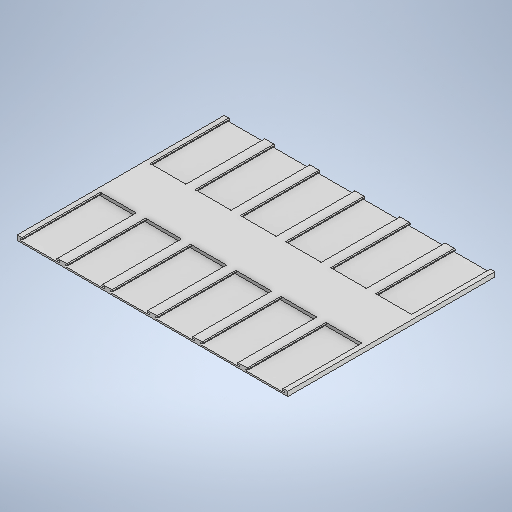
# Autodesk Inventor part: Holder
Saved by Autodesk Inventor 2025 (Build 290162000, 162)
## iProperties
Created: 2025-01-15
Part Number: Holder
Material: Generic
Document SubType Name: Modeling
Designer: ethan
Density: 1 g/cm^3
Appearance: Default
Author: ethan
Autodesk Inventor part; units mm, degrees
ref_plane "YZ Plane" through (0, 0, 0) normal (1, 0, 0) x (0, 1, 0)
ref_plane "XZ Plane" through (0, 0, 0) normal (0, 1, 0) x (-1, 0, 0)
ref_plane "XY Plane" through (0, 0, 0) normal (0, 0, 1) x (1, 0, 0)
sketch "Sketch1" plane through (0, 0, 0) normal (0, 1, 0) x (-1, 0, 0)
  line L0 (0, 0) -> (25.4, 0) construction
  line L1 (25.4, 0) -> (25.4, -50.8) construction
  line L2 (25.4, -50.8) -> (0, -50.8) construction
  line L3 (0, -50.8) -> (0, 0) construction
  line L4 (23.9, -49.3) -> (23.9, -1.5) construction
  line L5 (23.9, -1.5) -> (1.5, -1.5) construction
  line L6 (1.5, -1.5) -> (1.5, -49.3) construction
  line L7 (1.5, -49.3) -> (23.9, -49.3) construction
  line L8 (0, 0) -> (-4, 0) construction
  line L9 (-29.4, 0) -> (-4, 0) construction
  line L10 (-4, 0) -> (-4, -50.8) construction
  line L11 (-4, -50.8) -> (-29.4, -50.8) construction
  line L12 (-29.4, -50.8) -> (-29.4, 0) construction
  line L13 (-5.5, -49.3) -> (-5.5, -1.5) construction
  line L14 (-5.5, -1.5) -> (-27.9, -1.5) construction
  line L15 (-27.9, -1.5) -> (-27.9, -49.3) construction
  line L16 (-27.9, -49.3) -> (-5.5, -49.3) construction
  line L17 (-58.8, 0) -> (-33.4, 0) construction
  line L18 (-33.4, 0) -> (-33.4, -50.8) construction
  line L19 (-33.4, -50.8) -> (-58.8, -50.8) construction
  line L20 (-58.8, -50.8) -> (-58.8, 0) construction
  line L21 (-34.9, -49.3) -> (-34.9, -1.5) construction
  line L22 (-34.9, -1.5) -> (-57.3, -1.5) construction
  line L23 (-57.3, -1.5) -> (-57.3, -49.3) construction
  line L24 (-57.3, -49.3) -> (-34.9, -49.3) construction
  line L25 (-88.2, 0) -> (-62.8, 0) construction
  line L26 (-62.8, 0) -> (-62.8, -50.8) construction
  line L27 (-62.8, -50.8) -> (-88.2, -50.8) construction
  line L28 (-88.2, -50.8) -> (-88.2, 0) construction
  line L29 (-64.3, -49.3) -> (-64.3, -1.5) construction
  line L30 (-64.3, -1.5) -> (-86.7, -1.5) construction
  line L31 (-86.7, -1.5) -> (-86.7, -49.3) construction
  line L32 (-86.7, -49.3) -> (-64.3, -49.3) construction
  line L33 (-117.6, 0) -> (-92.2, 0) construction
  line L34 (-92.2, 0) -> (-92.2, -50.8) construction
  line L35 (-92.2, -50.8) -> (-117.6, -50.8) construction
  line L36 (-117.6, -50.8) -> (-117.6, 0) construction
  line L37 (-93.7, -49.3) -> (-93.7, -1.5) construction
  line L38 (-93.7, -1.5) -> (-116.1, -1.5) construction
  line L39 (-116.1, -1.5) -> (-116.1, -49.3) construction
  line L40 (-116.1, -49.3) -> (-93.7, -49.3) construction
  line L41 (-147, 0) -> (-121.6, 0) construction
  line L42 (-121.6, 0) -> (-121.6, -50.8) construction
  line L43 (-121.6, -50.8) -> (-147, -50.8) construction
  line L44 (-147, -50.8) -> (-147, 0) construction
  line L45 (-123.1, -49.3) -> (-123.1, -1.5) construction
  line L46 (-123.1, -1.5) -> (-145.5, -1.5) construction
  line L47 (-145.5, -1.5) -> (-145.5, -49.3) construction
  line L48 (-145.5, -49.3) -> (-123.1, -49.3) construction
  line L49 (0, 80.2) -> (25.4, 80.2) construction
  line L50 (25.4, 80.2) -> (25.4, 29.4) construction
  line L51 (25.4, 29.4) -> (0, 29.4) construction
  line L52 (0, 29.4) -> (0, 80.2) construction
  line L53 (23.9, 30.9) -> (23.9, 78.7) construction
  line L54 (23.9, 78.7) -> (1.5, 78.7) construction
  line L55 (1.5, 78.7) -> (1.5, 30.9) construction
  line L56 (1.5, 30.9) -> (23.9, 30.9) construction
  line L57 (-29.4, 80.2) -> (-4, 80.2) construction
  line L58 (-4, 80.2) -> (-4, 29.4) construction
  line L59 (-4, 29.4) -> (-29.4, 29.4) construction
  line L60 (-29.4, 29.4) -> (-29.4, 80.2) construction
  line L61 (-5.5, 30.9) -> (-5.5, 78.7) construction
  line L62 (-5.5, 78.7) -> (-27.9, 78.7) construction
  line L63 (-27.9, 78.7) -> (-27.9, 30.9) construction
  line L64 (-27.9, 30.9) -> (-5.5, 30.9) construction
  line L65 (-58.8, 80.2) -> (-33.4, 80.2) construction
  line L66 (-33.4, 80.2) -> (-33.4, 29.4) construction
  line L67 (-33.4, 29.4) -> (-58.8, 29.4) construction
  line L68 (-58.8, 29.4) -> (-58.8, 80.2) construction
  line L69 (-34.9, 30.9) -> (-34.9, 78.7) construction
  line L70 (-34.9, 78.7) -> (-57.3, 78.7) construction
  line L71 (-57.3, 78.7) -> (-57.3, 30.9) construction
  line L72 (-57.3, 30.9) -> (-34.9, 30.9) construction
  line L73 (-88.2, 80.2) -> (-62.8, 80.2) construction
  line L74 (-62.8, 80.2) -> (-62.8, 29.4) construction
  line L75 (-62.8, 29.4) -> (-88.2, 29.4) construction
  line L76 (-88.2, 29.4) -> (-88.2, 80.2) construction
  line L77 (-64.3, 30.9) -> (-64.3, 78.7) construction
  line L78 (-64.3, 78.7) -> (-86.7, 78.7) construction
  line L79 (-86.7, 78.7) -> (-86.7, 30.9) construction
  line L80 (-86.7, 30.9) -> (-64.3, 30.9) construction
  line L81 (-117.6, 80.2) -> (-92.2, 80.2) construction
  line L82 (-92.2, 80.2) -> (-92.2, 29.4) construction
  line L83 (-92.2, 29.4) -> (-117.6, 29.4) construction
  line L84 (-117.6, 29.4) -> (-117.6, 80.2) construction
  line L85 (-93.7, 30.9) -> (-93.7, 78.7) construction
  line L86 (-93.7, 78.7) -> (-116.1, 78.7) construction
  line L87 (-116.1, 78.7) -> (-116.1, 30.9) construction
  line L88 (-116.1, 30.9) -> (-93.7, 30.9) construction
  line L89 (-147, 80.2) -> (-121.6, 80.2) construction
  line L90 (-121.6, 80.2) -> (-121.6, 29.4) construction
  line L91 (-121.6, 29.4) -> (-147, 29.4) construction
  line L92 (-147, 29.4) -> (-147, 80.2) construction
  line L93 (-123.1, 30.9) -> (-123.1, 78.7) construction
  line L94 (-123.1, 78.7) -> (-145.5, 78.7) construction
  line L95 (-145.5, 78.7) -> (-145.5, 30.9) construction
  line L96 (-145.5, 30.9) -> (-123.1, 30.9) construction
  line L97 (25.4, -50.8) -> (27.4, -50.8) construction
  line L98 (27.4, -50.8) -> (27.4, -52.8) construction
  line L99 (27.4, -52.8) -> (25.4, -52.8) construction
  line L100 (25.4, -52.8) -> (25.4, -50.8) construction
  line L101 (-147, 80.2) -> (-149, 80.2) construction
  line L102 (-149, 80.2) -> (-149, 82.2) construction
  line L103 (-149, 82.2) -> (-147, 82.2) construction
  line L104 (-147, 82.2) -> (-147, 80.2) construction
  line L105 (27.4, -52.8) -> (-149, -52.8)
  line L106 (-149, -52.8) -> (-149, 82.2)
  line L107 (-149, 82.2) -> (27.4, 82.2)
  line L108 (27.4, 82.2) -> (27.4, -52.8)
  line L109 (23.9, 0) -> (27.4, 0)
  line L110 (27.4, 0) -> (27.4, -52.8)
  line L111 (27.4, -52.8) -> (23.9, -52.8)
  line L112 (23.9, -52.8) -> (23.9, 0)
  line L113 (-149, -49.3) -> (-149, -52.8)
  line L114 (-149, -52.8) -> (27.4, -52.8)
  line L115 (27.4, -52.8) -> (27.4, -49.3)
  line L116 (27.4, -1.5) -> (-149, -1.5)
  line L117 (-149, -1.5) -> (-149, 30.9)
  line L118 (-149, 30.9) -> (27.4, 30.9)
  line L119 (27.4, 30.9) -> (27.4, -1.5)
  line L120 (1.5, -1.5) -> (-5.5, -1.5)
  line L121 (-5.5, -1.5) -> (-5.5, -49.3)
  line L122 (-5.5, -49.3) -> (1.5, -49.3)
  line L123 (1.5, -49.3) -> (1.5, -1.5)
  line L124 (-27.9, -49.3) -> (-34.9, -49.3)
  line L125 (-34.9, -49.3) -> (-34.9, -1.5)
  line L126 (-34.9, -1.5) -> (-27.9, -1.5)
  line L127 (-27.9, -1.5) -> (-27.9, -49.3)
  line L128 (-57.3, -1.5) -> (-64.3, -1.5)
  line L129 (-64.3, -1.5) -> (-64.3, -49.3)
  line L130 (-64.3, -49.3) -> (-57.3, -49.3)
  line L131 (-57.3, -49.3) -> (-57.3, -1.5)
  line L132 (-86.7, -49.3) -> (-93.7, -49.3)
  line L133 (-93.7, -49.3) -> (-93.7, -1.5)
  line L134 (-93.7, -1.5) -> (-86.7, -1.5)
  line L135 (-86.7, -1.5) -> (-86.7, -49.3)
  line L136 (-116.1, -1.5) -> (-123.1, -1.5)
  line L137 (-123.1, -1.5) -> (-123.1, -49.3)
  line L138 (-123.1, -49.3) -> (-116.1, -49.3)
  line L139 (-116.1, -49.3) -> (-116.1, -1.5)
  line L140 (-145.5, -49.3) -> (-149, -49.3)
  line L141 (-149, -49.3) -> (-149, -1.5)
  line L142 (-149, -1.5) -> (-145.5, -1.5)
  line L143 (-145.5, -1.5) -> (-145.5, -49.3)
  line L144 (23.9, 30.9) -> (27.4, 30.9)
  line L145 (27.4, 30.9) -> (27.4, 78.7)
  line L146 (27.4, 78.7) -> (23.9, 78.7)
  line L147 (23.9, 78.7) -> (23.9, 30.9)
  line L148 (-149, 78.7) -> (-149, 82.2)
  line L149 (-149, 82.2) -> (27.4, 82.2)
  line L150 (27.4, 82.2) -> (27.4, 78.7)
  line L151 (-145.5, 30.9) -> (-149, 30.9)
  line L152 (-149, 30.9) -> (-149, 78.7)
  line L153 (-149, 78.7) -> (-145.5, 78.7)
  line L154 (-145.5, 78.7) -> (-145.5, 30.9)
  line L155 (-123.1, 78.7) -> (-116.1, 78.7)
  line L156 (-116.1, 78.7) -> (-116.1, 30.9)
  line L157 (-116.1, 30.9) -> (-123.1, 30.9)
  line L158 (-123.1, 30.9) -> (-123.1, 78.7)
  line L159 (-93.7, 30.9) -> (-86.7, 30.9)
  line L160 (-86.7, 30.9) -> (-86.7, 78.7)
  line L161 (-86.7, 78.7) -> (-93.7, 78.7)
  line L162 (-93.7, 78.7) -> (-93.7, 30.9)
  line L163 (-64.3, 78.7) -> (-57.3, 78.7)
  line L164 (-57.3, 78.7) -> (-57.3, 30.9)
  line L165 (-57.3, 30.9) -> (-64.3, 30.9)
  line L166 (-64.3, 30.9) -> (-64.3, 78.7)
  line L167 (-34.9, 30.9) -> (-27.9, 30.9)
  line L168 (-27.9, 30.9) -> (-27.9, 78.7)
  line L169 (-27.9, 78.7) -> (-34.9, 78.7)
  line L170 (-34.9, 78.7) -> (-34.9, 30.9)
  line L171 (-5.5, 78.7) -> (1.5, 78.7)
  line L172 (1.5, 78.7) -> (1.5, 30.9)
  line L173 (1.5, 30.9) -> (-5.5, 30.9)
  line L174 (-5.5, 30.9) -> (-5.5, 78.7)
  line L175 (-145.5, 78.7) -> (-149, 78.7)
  line L176 (-149, 78.7) -> (-149, 82.2)
  line L177 (-149, 82.2) -> (-145.5, 82.2)
  line L178 (-145.5, 82.2) -> (-145.5, 78.7)
  line L179 (-123.1, 78.7) -> (-116.1, 78.7)
  line L180 (-116.1, 78.7) -> (-116.1, 82.2)
  line L181 (-116.1, 82.2) -> (-123.1, 82.2)
  line L182 (-123.1, 82.2) -> (-123.1, 78.7)
  line L183 (-93.7, 78.7) -> (-86.7, 78.7)
  line L184 (-86.7, 78.7) -> (-86.7, 82.2)
  line L185 (-86.7, 82.2) -> (-93.7, 82.2)
  line L186 (-93.7, 82.2) -> (-93.7, 78.7)
  line L187 (-64.3, 78.7) -> (-57.3, 78.7)
  line L188 (-57.3, 78.7) -> (-57.3, 82.2)
  line L189 (-57.3, 82.2) -> (-64.3, 82.2)
  line L190 (-64.3, 82.2) -> (-64.3, 78.7)
  line L191 (-34.9, 78.7) -> (-27.9, 78.7)
  line L192 (-27.9, 78.7) -> (-27.9, 82.2)
  line L193 (-27.9, 82.2) -> (-34.9, 82.2)
  line L194 (-34.9, 82.2) -> (-34.9, 78.7)
  line L195 (-5.5, 78.7) -> (1.5, 78.7)
  line L196 (1.5, 78.7) -> (1.5, 82.2)
  line L197 (1.5, 82.2) -> (-5.5, 82.2)
  line L198 (-5.5, 82.2) -> (-5.5, 78.7)
  line L199 (23.9, 78.7) -> (27.4, 78.7)
  line L200 (27.4, 78.7) -> (27.4, 82.2)
  line L201 (27.4, 82.2) -> (23.9, 82.2)
  line L202 (23.9, 82.2) -> (23.9, 78.7)
  line L203 (-145.5, -49.3) -> (-149, -49.3)
  line L204 (-149, -49.3) -> (-149, -52.8)
  line L205 (-149, -52.8) -> (-145.5, -52.8)
  line L206 (-145.5, -52.8) -> (-145.5, -49.3)
  line L207 (-123.1, -49.3) -> (-116.1, -49.3)
  line L208 (-116.1, -49.3) -> (-116.1, -52.8)
  line L209 (-116.1, -52.8) -> (-123.1, -52.8)
  line L210 (-123.1, -52.8) -> (-123.1, -49.3)
  line L211 (-93.7, -49.3) -> (-86.7, -49.3)
  line L212 (-86.7, -49.3) -> (-86.7, -52.8)
  line L213 (-86.7, -52.8) -> (-93.7, -52.8)
  line L214 (-93.7, -52.8) -> (-93.7, -49.3)
  line L215 (-64.3, -49.3) -> (-57.3, -49.3)
  line L216 (-57.3, -49.3) -> (-57.3, -52.8)
  line L217 (-57.3, -52.8) -> (-64.3, -52.8)
  line L218 (-64.3, -52.8) -> (-64.3, -49.3)
  line L219 (-34.9, -49.3) -> (-27.9, -49.3)
  line L220 (-27.9, -49.3) -> (-27.9, -52.8)
  line L221 (-27.9, -52.8) -> (-34.9, -52.8)
  line L222 (-34.9, -52.8) -> (-34.9, -49.3)
  line L223 (-5.5, -49.3) -> (1.5, -49.3)
  line L224 (1.5, -49.3) -> (1.5, -52.8)
  line L225 (1.5, -52.8) -> (-5.5, -52.8)
  line L226 (-5.5, -52.8) -> (-5.5, -49.3)
  point P0 (-93.7, -1.5)
  point P1 (-34.9, -1.5)
  point P2 (1.5, -49.3)
  point P3 (1.5, 78.7)
  dimension "d0" = 25.4
  dimension "d1" = 50.8
  dimension "d2" = 1.5
  dimension "d3" = 4
  dimension "d6" = 29.4
  dimension "d9" = 80.2
  dimension "d12" = 2
  dimension "d13" = 2
  dimension "d14" = 2
  dimension "d15" = 2
  constraints: 454 end point, 68 parallel, 34 horizontal, 33 perpendicular, 16 point on line, 1 collinear, 1 vertical, 178 other
  measures "d0" distance of L1.end L2.end
  measures "d1" distance of L0.end L1.end
  measures "d2" distance between parallel lines of L1 L4
  measures "d3" distance of L0.start L8.end
  measures "d6" distance of L0.start L9.start
  measures "d9" distance of L0.start L49.start
  measures "d12" distance of L98.end L99.end
  measures "d13" distance of L97.end L98.end
  measures "d14" distance of L102.end L103.end
  measures "d15" distance of L101.end L102.end
extrude "Extrusion1" add sketch "Sketch1" along normal blind 1 contours L105 L112 L116 L108 | L105 L226 L122 L224 | L116 L106 L118 L108 L109 L112 | L112 L109 L108 L116 | L122 L121 L116 L123 | L105 L222 L124 L220 | L118 L147 L146 L108 | L124 L125 L116 L127 | L146 L202 L107 L108 | L105 L218 L130 L216 | L118 L174 L171 L172 | L130 L129 L116 L131 | L171 L198 L107 L196 | L105 L214 L132 L212 | L118 L170 L169 L168 | L132 L133 L116 L135 | L169 L194 L107 L192 | L105 L210 L138 L208 | L118 L166 L163 L164 | L138 L137 L116 L139 | L163 L190 L107 L188 | L105 L106 L140 L206 | L118 L162 L161 L160 | L140 L106 L116 L143 | L161 L186 L107 L184 | L118 L158 L155 L156 | L106 L153 L154 L118 | L155 L182 L107 L180 | L106 L107 L178 L153
sketch "Sketch2" plane through (0, 0, 0) normal (0, -1, 0) x (1, 0, 0)
  line L0 (149, -52.8) -> (145.5, -52.8) construction
  line L1 (149, 82.2) -> (149, -52.8) construction
  line L2 (145.5, 82.2) -> (149, 82.2) construction
  line L3 (145.5, 30.9) -> (145.5, 82.2) construction
  line L4 (123.1, 30.9) -> (145.5, 30.9) construction
  line L5 (123.1, 82.2) -> (123.1, 30.9) construction
  line L6 (116.1, 82.2) -> (123.1, 82.2) construction
  line L7 (116.1, 30.9) -> (116.1, 82.2) construction
  line L8 (93.7, 30.9) -> (116.1, 30.9) construction
  line L9 (93.7, 82.2) -> (93.7, 30.9) construction
  line L10 (86.7, 82.2) -> (93.7, 82.2) construction
  line L11 (86.7, 30.9) -> (86.7, 82.2) construction
  line L12 (64.3, 30.9) -> (86.7, 30.9) construction
  line L13 (64.3, 82.2) -> (64.3, 30.9) construction
  line L14 (57.3, 82.2) -> (64.3, 82.2) construction
  line L15 (57.3, 30.9) -> (57.3, 82.2) construction
  line L16 (34.9, 30.9) -> (57.3, 30.9) construction
  line L17 (34.9, 82.2) -> (34.9, 30.9) construction
  line L18 (27.9, 82.2) -> (34.9, 82.2) construction
  line L19 (27.9, 30.9) -> (27.9, 82.2) construction
  line L20 (5.5, 30.9) -> (27.9, 30.9) construction
  line L21 (5.5, 82.2) -> (5.5, 30.9) construction
  line L22 (-1.5, 82.2) -> (5.5, 82.2) construction
  line L23 (-1.5, 30.9) -> (-1.5, 82.2) construction
  line L24 (-23.9, 30.9) -> (-1.5, 30.9) construction
  line L25 (-23.9, 82.2) -> (-23.9, 30.9) construction
  line L26 (-27.4, 82.2) -> (-23.9, 82.2) construction
  line L27 (-27.4, -52.8) -> (-27.4, 82.2) construction
  line L28 (-23.9, -52.8) -> (-27.4, -52.8) construction
  line L29 (-23.9, -1.5) -> (-23.9, -52.8) construction
  line L30 (-1.5, -1.5) -> (-23.9, -1.5) construction
  line L31 (-1.5, -52.8) -> (-1.5, -1.5) construction
  line L32 (5.5, -52.8) -> (-1.5, -52.8) construction
  line L33 (5.5, -1.5) -> (5.5, -52.8) construction
  line L34 (27.9, -1.5) -> (5.5, -1.5) construction
  line L35 (27.9, -52.8) -> (27.9, -1.5) construction
  line L36 (34.9, -52.8) -> (27.9, -52.8) construction
  line L37 (34.9, -1.5) -> (34.9, -52.8) construction
  line L38 (57.3, -1.5) -> (34.9, -1.5) construction
  line L39 (57.3, -52.8) -> (57.3, -1.5) construction
  line L40 (64.3, -52.8) -> (57.3, -52.8) construction
  line L41 (64.3, -1.5) -> (64.3, -52.8) construction
  line L42 (86.7, -1.5) -> (64.3, -1.5) construction
  line L43 (86.7, -52.8) -> (86.7, -1.5) construction
  line L44 (93.7, -52.8) -> (86.7, -52.8) construction
  line L45 (93.7, -1.5) -> (93.7, -52.8) construction
  line L46 (116.1, -1.5) -> (93.7, -1.5) construction
  line L47 (116.1, -52.8) -> (116.1, -1.5) construction
  line L48 (123.1, -52.8) -> (116.1, -52.8) construction
  line L49 (123.1, -1.5) -> (123.1, -52.8) construction
  line L50 (145.5, -1.5) -> (123.1, -1.5) construction
  line L51 (145.5, -52.8) -> (145.5, -1.5) construction
  line L52 (147, 0) -> (121.6, 0) construction
  line L53 (121.6, 0) -> (121.6, -51.3) construction
  line L54 (121.6, -51.3) -> (117.6, -51.3) construction
  line L55 (117.6, -51.3) -> (117.6, 0) construction
  line L56 (117.6, 0) -> (92.2, 0) construction
  line L57 (92.2, 0) -> (92.2, -51.3) construction
  line L58 (92.2, -51.3) -> (88.2, -51.3) construction
  line L59 (88.2, -51.3) -> (88.2, 0) construction
  line L60 (88.2, 0) -> (62.8, 0) construction
  line L61 (62.8, 0) -> (62.8, -51.3) construction
  line L62 (62.8, -51.3) -> (58.8, -51.3) construction
  line L63 (58.8, -51.3) -> (58.8, 0) construction
  line L64 (58.8, 0) -> (33.4, 0) construction
  line L65 (33.4, 0) -> (33.4, -51.3) construction
  line L66 (33.4, -51.3) -> (29.4, -51.3) construction
  line L67 (29.4, -51.3) -> (29.4, 0) construction
  line L68 (29.4, 0) -> (4, 0) construction
  line L69 (4, 0) -> (4, -51.3) construction
  line L70 (4, -51.3) -> (0, -51.3) construction
  line L71 (0, -51.3) -> (0, 0) construction
  line L72 (0, 0) -> (-25.4, 0) construction
  line L73 (-25.4, 0) -> (-25.4, -51.3) construction
  line L74 (-25.4, -51.3) -> (-25.9, -51.3) construction
  line L75 (-25.9, -51.3) -> (-25.9, 80.7) construction
  line L76 (-25.9, 80.7) -> (-25.4, 80.7) construction
  line L77 (-25.4, 80.7) -> (-25.4, 29.4) construction
  line L78 (-25.4, 29.4) -> (0, 29.4) construction
  line L79 (0, 29.4) -> (0, 80.7) construction
  line L80 (0, 80.7) -> (4, 80.7) construction
  line L81 (4, 80.7) -> (4, 29.4) construction
  line L82 (4, 29.4) -> (29.4, 29.4) construction
  line L83 (29.4, 29.4) -> (29.4, 80.7) construction
  line L84 (29.4, 80.7) -> (33.4, 80.7) construction
  line L85 (33.4, 80.7) -> (33.4, 29.4) construction
  line L86 (33.4, 29.4) -> (58.8, 29.4) construction
  line L87 (58.8, 29.4) -> (58.8, 80.7) construction
  line L88 (58.8, 80.7) -> (62.8, 80.7) construction
  line L89 (62.8, 80.7) -> (62.8, 29.4) construction
  line L90 (62.8, 29.4) -> (88.2, 29.4) construction
  line L91 (88.2, 29.4) -> (88.2, 80.7) construction
  line L92 (88.2, 80.7) -> (92.2, 80.7) construction
  line L93 (92.2, 80.7) -> (92.2, 29.4) construction
  line L94 (92.2, 29.4) -> (117.6, 29.4) construction
  line L95 (117.6, 29.4) -> (117.6, 80.7) construction
  line L96 (117.6, 80.7) -> (121.6, 80.7) construction
  line L97 (121.6, 80.7) -> (121.6, 29.4) construction
  line L98 (121.6, 29.4) -> (147, 29.4) construction
  line L99 (147, 29.4) -> (147, 80.7) construction
  line L100 (147, 80.7) -> (147.5, 80.7) construction
  line L101 (147.5, 80.7) -> (147.5, -51.3) construction
  line L102 (147.5, -51.3) -> (147, -51.3) construction
  line L103 (147, -51.3) -> (147, 0) construction
  line L104 (147, -51.3) -> (147, -52.8)
  line L105 (149, -52.8) -> (145.5, -52.8) projected
  line L106 (147, -52.8) -> (149, -52.8)
  line L107 (149, -52.8) -> (149, 82.2)
  line L108 (147, 82.2) -> (149, 82.2)
  line L109 (147, 82.2) -> (147, 29.4)
  line L110 (147, 29.4) -> (121.6, 29.4)
  line L111 (121.6, 29.4) -> (121.6, 82.2)
  line L112 (121.6, 82.2) -> (117.6, 82.2)
  line L113 (117.6, 82.2) -> (117.6, 29.4)
  line L114 (117.6, 29.4) -> (92.2, 29.4)
  line L115 (88.2, 29.4) -> (62.8, 29.4)
  line L116 (58.8, 29.4) -> (33.4, 29.4)
  line L117 (29.4, 29.4) -> (4, 29.4)
  line L118 (0, 29.4) -> (-25.4, 29.4)
  line L119 (92.2, 29.4) -> (92.2, 82.2)
  line L120 (92.2, 82.2) -> (88.2, 82.2)
  line L121 (88.2, 82.2) -> (88.2, 29.4)
  line L122 (62.8, 29.4) -> (62.8, 82.2)
  line L123 (62.8, 82.2) -> (58.8, 82.2)
  line L124 (58.8, 82.2) -> (58.8, 29.4)
  line L125 (33.4, 29.4) -> (33.4, 82.2)
  line L126 (33.4, 82.2) -> (29.4, 82.2)
  line L127 (29.4, 82.2) -> (29.4, 29.4)
  line L128 (4, 29.4) -> (4, 82.2)
  line L129 (4, 82.2) -> (0, 82.2)
  line L130 (0, 82.2) -> (0, 29.4)
  line L131 (-25.4, 29.4) -> (-25.4, 82.2)
  line L132 (-25.4, 82.2) -> (-27.4, 82.2)
  line L133 (-27.4, 82.2) -> (-27.4, -52.8)
  line L134 (149, 14.7) -> (-27.4, 14.7) construction
  line L135 (145.5, -52.8) -> (149, -52.8) construction
  line L136 (145.5, -1.5) -> (145.5, -52.8) construction
  line L137 (123.1, -1.5) -> (145.5, -1.5) construction
  line L138 (123.1, -52.8) -> (123.1, -1.5) construction
  line L139 (116.1, -52.8) -> (123.1, -52.8) construction
  line L140 (116.1, -1.5) -> (116.1, -52.8) construction
  line L141 (93.7, -1.5) -> (116.1, -1.5) construction
  line L142 (93.7, -52.8) -> (93.7, -1.5) construction
  line L143 (86.7, -52.8) -> (93.7, -52.8) construction
  line L144 (86.7, -1.5) -> (86.7, -52.8) construction
  line L145 (64.3, -1.5) -> (86.7, -1.5) construction
  line L146 (64.3, -52.8) -> (64.3, -1.5) construction
  line L147 (57.3, -52.8) -> (64.3, -52.8) construction
  line L148 (57.3, -1.5) -> (57.3, -52.8) construction
  line L149 (34.9, -1.5) -> (57.3, -1.5) construction
  line L150 (34.9, -52.8) -> (34.9, -1.5) construction
  line L151 (27.9, -52.8) -> (34.9, -52.8) construction
  line L152 (27.9, -1.5) -> (27.9, -52.8) construction
  line L153 (5.5, -1.5) -> (27.9, -1.5) construction
  line L154 (5.5, -52.8) -> (5.5, -1.5) construction
  line L155 (-1.5, -52.8) -> (5.5, -52.8) construction
  line L156 (-1.5, -1.5) -> (-1.5, -52.8) construction
  line L157 (-23.9, -1.5) -> (-1.5, -1.5) construction
  line L158 (-23.9, -52.8) -> (-23.9, -1.5) construction
  line L159 (-27.4, -52.8) -> (-23.9, -52.8) construction
  line L160 (-25.9, -51.3) -> (-25.4, -51.3) construction
  line L161 (-25.4, -51.3) -> (-25.4, 0) construction
  line L162 (-25.4, 0) -> (0, 0) construction
  line L163 (0, 0) -> (0, -51.3) construction
  line L164 (0, -51.3) -> (4, -51.3) construction
  line L165 (4, -51.3) -> (4, 0) construction
  line L166 (4, 0) -> (29.4, 0) construction
  line L167 (29.4, 0) -> (29.4, -51.3) construction
  line L168 (29.4, -51.3) -> (33.4, -51.3) construction
  line L169 (33.4, -51.3) -> (33.4, 0) construction
  line L170 (33.4, 0) -> (58.8, 0) construction
  line L171 (58.8, 0) -> (58.8, -51.3) construction
  line L172 (58.8, -51.3) -> (62.8, -51.3) construction
  line L173 (62.8, -51.3) -> (62.8, 0) construction
  line L174 (62.8, 0) -> (88.2, 0) construction
  line L175 (88.2, 0) -> (88.2, -51.3) construction
  line L176 (88.2, -51.3) -> (92.2, -51.3) construction
  line L177 (92.2, -51.3) -> (92.2, 0) construction
  line L178 (92.2, 0) -> (117.6, 0) construction
  line L179 (117.6, 0) -> (117.6, -51.3) construction
  line L180 (117.6, -51.3) -> (121.6, -51.3) construction
  line L181 (121.6, -51.3) -> (121.6, 0) construction
  line L182 (121.6, 0) -> (147, 0) construction
  line L183 (147, 0) -> (147, -51.3) construction
  line L184 (147, -51.3) -> (147.5, -51.3) construction
  line L185 (147, -52.8) -> (149, -52.8)
  line L186 (147, -52.8) -> (147, 0)
  line L187 (147, 0) -> (121.6, 0)
  line L188 (121.6, 0) -> (121.6, -52.8)
  line L189 (121.6, -52.8) -> (117.6, -52.8)
  line L190 (117.6, -52.8) -> (117.6, 0)
  line L191 (117.6, 0) -> (92.2, 0)
  line L192 (88.2, 0) -> (62.8, 0)
  line L193 (58.8, 0) -> (33.4, 0)
  line L194 (29.4, 0) -> (4, 0)
  line L195 (0, 0) -> (-25.4, 0)
  line L196 (92.2, 0) -> (92.2, -52.8)
  line L197 (92.2, -52.8) -> (88.2, -52.8)
  line L198 (88.2, -52.8) -> (88.2, 0)
  line L199 (62.8, 0) -> (62.8, -52.8)
  line L200 (62.8, -52.8) -> (58.8, -52.8)
  line L201 (58.8, -52.8) -> (58.8, 0)
  line L202 (33.4, 0) -> (33.4, -52.8)
  line L203 (33.4, -52.8) -> (29.4, -52.8)
  line L204 (29.4, -52.8) -> (29.4, 0)
  line L205 (4, 0) -> (4, -52.8)
  line L206 (4, -52.8) -> (0, -52.8)
  line L207 (0, -52.8) -> (0, 0)
  line L208 (-25.4, 0) -> (-25.4, -52.8)
  line L209 (-25.4, -52.8) -> (-27.4, -52.8)
  point P0 (0, 0)
  dimension "d18" = 1.5
  constraints: 314 end point, 27 point on line, 13 collinear, 11 symmetric about line, 7 perpendicular, 2 midpoint, 2 parallel, 1 vertical, 51 other
  measures "d18" distance between parallel lines of L51 L103
extrude "Extrusion2" add sketch "Sketch2" along normal blind 1
sketch "Sketch3" plane through (0, -1, 0) normal (0, -1, 0) x (1, 0, 0)
  line L0 (149, 82.2) -> (147, 82.2) construction
  line L1 (147, 82.2) -> (147, 29.4) construction
  line L2 (147, 29.4) -> (121.6, 29.4) construction
  line L3 (121.6, 29.4) -> (121.6, 82.2) construction
  line L4 (121.6, 82.2) -> (117.6, 82.2) construction
  line L5 (117.6, 82.2) -> (117.6, 29.4) construction
  line L6 (117.6, 29.4) -> (92.2, 29.4) construction
  line L7 (92.2, 29.4) -> (92.2, 82.2) construction
  line L8 (92.2, 82.2) -> (88.2, 82.2) construction
  line L9 (88.2, 82.2) -> (88.2, 29.4) construction
  line L10 (88.2, 29.4) -> (62.8, 29.4) construction
  line L11 (62.8, 29.4) -> (62.8, 82.2) construction
  line L12 (62.8, 82.2) -> (58.8, 82.2) construction
  line L13 (58.8, 82.2) -> (58.8, 29.4) construction
  line L14 (58.8, 29.4) -> (33.4, 29.4) construction
  line L15 (33.4, 29.4) -> (33.4, 82.2) construction
  line L16 (33.4, 82.2) -> (29.4, 82.2) construction
  line L17 (29.4, 82.2) -> (29.4, 29.4) construction
  line L18 (29.4, 29.4) -> (4, 29.4) construction
  line L19 (4, 29.4) -> (4, 82.2) construction
  line L20 (4, 82.2) -> (0, 82.2) construction
  line L21 (0, 82.2) -> (0, 29.4) construction
  line L22 (0, 29.4) -> (-25.4, 29.4) construction
  line L23 (-25.4, 29.4) -> (-25.4, 82.2) construction
  line L24 (-25.4, 82.2) -> (-27.4, 82.2) construction
  line L25 (-27.4, 82.2) -> (-27.4, -52.8) construction
  line L26 (-27.4, -52.8) -> (-25.4, -52.8) construction
  line L27 (-25.4, -52.8) -> (-25.4, 0) construction
  line L28 (-25.4, 0) -> (0, 0) construction
  line L29 (0, 0) -> (0, -52.8) construction
  line L30 (0, -52.8) -> (4, -52.8) construction
  line L31 (4, -52.8) -> (4, 0) construction
  line L32 (4, 0) -> (29.4, 0) construction
  line L33 (29.4, 0) -> (29.4, -52.8) construction
  line L34 (29.4, -52.8) -> (33.4, -52.8) construction
  line L35 (33.4, -52.8) -> (33.4, 0) construction
  line L36 (33.4, 0) -> (58.8, 0) construction
  line L37 (58.8, 0) -> (58.8, -52.8) construction
  line L38 (58.8, -52.8) -> (62.8, -52.8) construction
  line L39 (62.8, -52.8) -> (62.8, 0) construction
  line L40 (62.8, 0) -> (88.2, 0) construction
  line L41 (88.2, 0) -> (88.2, -52.8) construction
  line L42 (88.2, -52.8) -> (92.2, -52.8) construction
  line L43 (92.2, -52.8) -> (92.2, 0) construction
  line L44 (92.2, 0) -> (117.6, 0) construction
  line L45 (117.6, 0) -> (117.6, -52.8) construction
  line L46 (117.6, -52.8) -> (121.6, -52.8) construction
  line L47 (121.6, -52.8) -> (121.6, 0) construction
  line L48 (121.6, 0) -> (147, 0) construction
  line L49 (147, 0) -> (147, -52.8) construction
  line L50 (147, -52.8) -> (149, -52.8) construction
  line L51 (149, -52.8) -> (149, 82.2) construction
  line L52 (149, -52.8) -> (-27.4, -52.8)
  line L53 (-27.4, -52.8) -> (-27.4, 82.2)
  line L54 (-27.4, 82.2) -> (149, 82.2)
  line L55 (149, 82.2) -> (149, -52.8)
  point P0 (0, 0)
  constraints: 8 end point, 2 parallel, 1 horizontal, 1 perpendicular
extrude "Extrusion3" add sketch "Sketch3" along normal blind 1
sketch "Sketch4" plane through (0, -1, 0) normal (0, 1, 0) x (1, 0, 0)
  line L0 (0, 0) -> (0, 52.8) construction
  line L1 (-25.4, 52.8) -> (0, 52.8) construction
  line L2 (-25.4, 52.8) -> (-25.4, 0) construction
  line L3 (-25.4, 0) -> (0, 0) construction
  line L4 (4, 52.8) -> (4, 0) construction
  line L5 (4, 0) -> (29.4, 0) construction
  line L6 (29.4, 0) -> (29.4, 52.8) construction
  line L7 (4, 52.8) -> (29.4, 52.8) construction
  line L8 (33.4, 52.8) -> (33.4, 0) construction
  line L9 (33.4, 0) -> (58.8, 0) construction
  line L10 (58.8, 0) -> (58.8, 52.8) construction
  line L11 (33.4, 52.8) -> (58.8, 52.8) construction
  line L12 (62.8, 52.8) -> (62.8, 0) construction
  line L13 (62.8, 0) -> (88.2, 0) construction
  line L14 (88.2, 0) -> (88.2, 52.8) construction
  line L15 (62.8, 52.8) -> (88.2, 52.8) construction
  line L16 (92.2, 52.8) -> (92.2, 0) construction
  line L17 (92.2, 0) -> (117.6, 0) construction
  line L18 (117.6, 0) -> (117.6, 52.8) construction
  line L19 (92.2, 52.8) -> (117.6, 52.8) construction
  line L20 (121.6, 52.8) -> (121.6, 0) construction
  line L21 (121.6, 0) -> (147, 0) construction
  line L22 (147, 0) -> (147, 52.8) construction
  line L23 (121.6, 52.8) -> (147, 52.8) construction
  line L24 (147, -82.2) -> (147, -29.4) construction
  line L25 (147, -29.4) -> (121.6, -29.4) construction
  line L26 (121.6, -29.4) -> (121.6, -82.2) construction
  line L27 (147, -82.2) -> (121.6, -82.2) construction
  line L28 (92.2, -29.4) -> (92.2, -82.2) construction
  line L29 (117.6, -82.2) -> (92.2, -82.2) construction
  line L30 (117.6, -82.2) -> (117.6, -29.4) construction
  line L31 (117.6, -29.4) -> (92.2, -29.4) construction
  line L32 (62.8, -29.4) -> (62.8, -82.2) construction
  line L33 (88.2, -82.2) -> (62.8, -82.2) construction
  line L34 (88.2, -82.2) -> (88.2, -29.4) construction
  line L35 (88.2, -29.4) -> (62.8, -29.4) construction
  line L36 (33.4, -29.4) -> (33.4, -82.2) construction
  line L37 (58.8, -82.2) -> (33.4, -82.2) construction
  line L38 (58.8, -82.2) -> (58.8, -29.4) construction
  line L39 (58.8, -29.4) -> (33.4, -29.4) construction
  line L40 (4, -29.4) -> (4, -82.2) construction
  line L41 (29.4, -82.2) -> (4, -82.2) construction
  line L42 (29.4, -82.2) -> (29.4, -29.4) construction
  line L43 (29.4, -29.4) -> (4, -29.4) construction
  line L44 (-25.4, -29.4) -> (-25.4, -82.2) construction
  line L45 (0, -82.2) -> (-25.4, -82.2) construction
  line L46 (0, -82.2) -> (0, -29.4) construction
  line L47 (0, -29.4) -> (-25.4, -29.4) construction
  line L48 (149, 52.8) -> (145.5, 52.8) construction
  line L49 (145.5, 52.8) -> (145.5, 1.5) construction
  line L50 (145.5, 1.5) -> (123.1, 1.5) construction
  line L51 (123.1, 1.5) -> (123.1, 52.8) construction
  line L52 (123.1, 52.8) -> (116.1, 52.8) construction
  line L53 (116.1, 52.8) -> (116.1, 1.5) construction
  line L54 (116.1, 1.5) -> (93.7, 1.5) construction
  line L55 (93.7, 1.5) -> (93.7, 52.8) construction
  line L56 (93.7, 52.8) -> (86.7, 52.8) construction
  line L57 (86.7, 52.8) -> (86.7, 1.5) construction
  line L58 (86.7, 1.5) -> (64.3, 1.5) construction
  line L59 (64.3, 1.5) -> (64.3, 52.8) construction
  line L60 (64.3, 52.8) -> (57.3, 52.8) construction
  line L61 (57.3, 52.8) -> (57.3, 1.5) construction
  line L62 (57.3, 1.5) -> (34.9, 1.5) construction
  line L63 (34.9, 1.5) -> (34.9, 52.8) construction
  line L64 (34.9, 52.8) -> (27.9, 52.8) construction
  line L65 (27.9, 52.8) -> (27.9, 1.5) construction
  line L66 (27.9, 1.5) -> (5.5, 1.5) construction
  line L67 (5.5, 1.5) -> (5.5, 52.8) construction
  line L68 (5.5, 52.8) -> (-1.5, 52.8) construction
  line L69 (-1.5, 52.8) -> (-1.5, 1.5) construction
  line L70 (-1.5, 1.5) -> (-23.9, 1.5) construction
  line L71 (-23.9, 1.5) -> (-23.9, 52.8) construction
  line L72 (-23.9, 52.8) -> (-27.4, 52.8) construction
  line L73 (-27.4, 52.8) -> (-27.4, -82.2) construction
  line L74 (-27.4, -82.2) -> (-23.9, -82.2) construction
  line L75 (-23.9, -82.2) -> (-23.9, -30.9) construction
  line L76 (-23.9, -30.9) -> (-1.5, -30.9) construction
  line L77 (-1.5, -30.9) -> (-1.5, -82.2) construction
  line L78 (-1.5, -82.2) -> (5.5, -82.2) construction
  line L79 (5.5, -82.2) -> (5.5, -30.9) construction
  line L80 (5.5, -30.9) -> (27.9, -30.9) construction
  line L81 (27.9, -30.9) -> (27.9, -82.2) construction
  line L82 (27.9, -82.2) -> (34.9, -82.2) construction
  line L83 (34.9, -82.2) -> (34.9, -30.9) construction
  line L84 (34.9, -30.9) -> (57.3, -30.9) construction
  line L85 (57.3, -30.9) -> (57.3, -82.2) construction
  line L86 (57.3, -82.2) -> (64.3, -82.2) construction
  line L87 (64.3, -82.2) -> (64.3, -30.9) construction
  line L88 (64.3, -30.9) -> (86.7, -30.9) construction
  line L89 (86.7, -30.9) -> (86.7, -82.2) construction
  line L90 (86.7, -82.2) -> (93.7, -82.2) construction
  line L91 (93.7, -82.2) -> (93.7, -30.9) construction
  line L92 (93.7, -30.9) -> (116.1, -30.9) construction
  line L93 (116.1, -30.9) -> (116.1, -82.2) construction
  line L94 (116.1, -82.2) -> (123.1, -82.2) construction
  line L95 (123.1, -82.2) -> (123.1, -30.9) construction
  line L96 (123.1, -30.9) -> (145.5, -30.9) construction
  line L97 (145.5, -30.9) -> (145.5, -82.2) construction
  line L98 (145.5, -82.2) -> (149, -82.2) construction
  line L99 (149, -82.2) -> (149, 52.8) construction
  line L100 (-25.4, -30.9) -> (147, -30.9) construction
  line L101 (147, -30.9) -> (147, 1.5) construction
  line L102 (147, 1.5) -> (-25.4, 1.5) construction
  line L103 (-25.4, 1.5) -> (-25.4, -30.9) construction
  line L104 (147, 1.5) -> (-25.4, 1.5)
  line L105 (-25.4, 1.5) -> (-25.4, -30.9)
  line L106 (-25.4, -30.9) -> (147, -30.9)
  line L107 (147, -30.9) -> (147, 1.5)
  point P0 (0, 0)
  constraints: 16 end point, 4 parallel, 2 horizontal, 2 perpendicular, 2 point on line
extrude "Extrusion4" add sketch "Sketch4" along normal blind 1
fillet "Fillet1" radius 0.5 24 edges at (-23.9, 1, -27.15) (-1.5, 1, -27.15) (5.5, 1, -27.15) (27.9, 1, -27.15) (34.9, 1, -27.15) (57.3, 1, -27.15) (64.3, 1, -27.15) (86.7, 1, -27.15) (93.7, 1, -27.15) (116.1, 1, -27.15) (123.1, 1, -27.15) (145.5, 1, -27.15) (145.5, 1, 56.55) (123.1, 1, 56.55) (116.1, 1, 56.55) (93.7, 1, 56.55) (86.7, 1, 56.55) (64.3, 1, 56.55) (57.3, 1, 56.55) (34.9, 1, 56.55) (27.9, 1, 56.55) (5.5, 1, 56.55) (-23.9, 1, 56.55) (-1.5, 1, 56.55)
body "Solid1"
